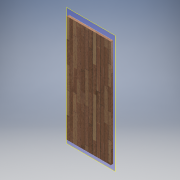
# Autodesk Inventor part: Vidrio
Saved by Autodesk Inventor 2018 (Build 220112000, 112)
## iProperties
Created: 2018-06-24
Part Number: Vidrio
Material: Wood (Maple)
Document SubType Name: Modeling
Designer: sebas
Density: 0.67 g/cm^3
Appearance: Natural Maple - Glossy Dark Tint
Author: sebas
Autodesk Inventor part; units mm, degrees
ref_plane "YZ Plane" through (0, 0, 0) normal (1, 0, 0) x (0, 1, 0)
ref_plane "XZ Plane" through (0, 0, 0) normal (0, 1, 0) x (-1, 0, 0)
ref_plane "XY Plane" through (0, 0, 0) normal (0, 0, 1) x (1, 0, 0)
sketch "Sketch1" plane through (0, 0, 0) normal (0, 1, 0) x (-1, 0, 0)
  line L0 (0, 0) -> (-651, 0)
  line L1 (-651, 0) -> (-651, 1582)
  line L2 (-651, 1582) -> (0, 1582)
  line L3 (0, 1582) -> (0, 0)
  dimension "TablaLargo" = 1582
  dimension "TablaProfundo" = 651
  constraints: 8 end point, 2 parallel, 1 horizontal, 1 perpendicular
  measures "TablaLargo" distance of L2.end L0.start
  measures "TablaProfundo" distance of L0.start L0.end
extrude "Madera" add sketch "Sketch1" along normal blind 30
ref_plane "Work Plane1" through (0, 30.1, 0) normal (0, 1, 0) x (1, 0, 0)
sketch "Sketch3" plane through (0, 30.1, 0) normal (0, 1, 0) x (1, 0, 0)
  line L0 (0, -1582) -> (651, -1582) projected
  line L1 (0, 0) -> (651, 0)
  line L2 (651, 0) -> (651, -1582)
  line L3 (651, -1582) -> (0, -1582)
  line L4 (0, -1582) -> (0, 0)
  constraints: 8 end point, 2 parallel, 1 horizontal, 1 perpendicular
extrude "Vidrio" add sketch "Sketch3" along normal blind 4
body "Solid1"
